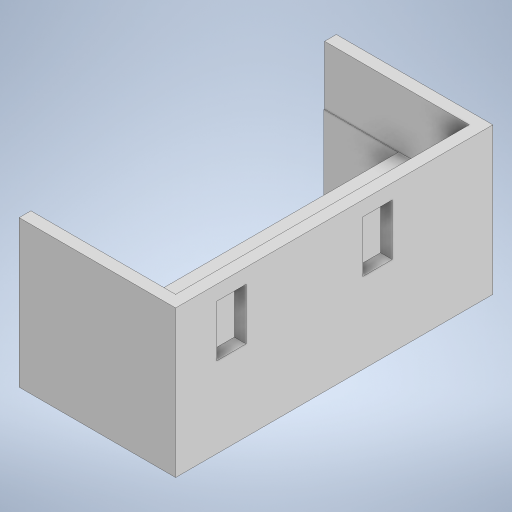
# Autodesk Inventor part: Base1
Saved by Autodesk Inventor 2023 (Build 270158000, 158)
## iProperties
Created: 2022-05-16
Part Number: Base1
Material: Generic
Document SubType Name: Modeling
Designer: WMGWW
Density: 1 g/cm^3
Appearance: Default
Author: WMGWW
Autodesk Inventor part; units mm, degrees
ref_plane "YZ Plane" through (0, 0, 0) normal (1, 0, 0) x (0, 1, 0)
ref_plane "XZ Plane" through (0, 0, 0) normal (0, 1, 0) x (-1, 0, 0)
ref_plane "XY Plane" through (0, 0, 0) normal (0, 0, 1) x (1, 0, 0)
sketch "Sketch1" plane through (0, 0, 0) normal (0, 1, 0) x (-1, 0, 0)
  line L0 (0, 0) -> (25.4, 0)
  line L1 (25.4, 0) -> (25.4, -127)
  line L2 (25.4, -127) -> (0, -127)
  line L3 (0, -127) -> (0, 0)
  line L4 (30.48, 5.08) -> (-5.08, 5.08)
  line L5 (-5.08, 5.08) -> (-5.08, -132.08)
  line L6 (-5.08, -132.08) -> (30.48, -132.08)
  line L7 (30.48, -132.08) -> (30.48, 5.08)
  dimension "d0" = 25.4
  dimension "d1" = 127
  dimension "d2" = 5.08
  dimension "d3" = 5.08
  dimension "d4" = 5.08
  dimension "d5" = 5.08
  constraints: 16 end point, 4 parallel, 2 horizontal, 2 perpendicular
  measures "d0" distance of L0.start L0.end
  measures "d1" distance of L0.end L1.end
  measures "d2" distance between parallel lines of L4 L0
  measures "d3" distance between parallel lines of L6 L2
  measures "d4" distance between parallel lines of L3 L5
  measures "d5" distance between parallel lines of L7 L1
extrude "Extrusion1" add sketch "Sketch1" along normal blind 38.1
sketch "Sketch2" plane through (0, 38.1, 0) normal (0, 1, 0) x (1, 0, 0)
  line L0 (-30.48, -5.08) -> (5.08, -5.08) projected
  line L1 (5.08, -5.08) -> (-62.5812, -5.08)
  line L2 (-62.5812, -5.08) -> (-62.5812, 0)
  line L3 (-62.5812, 0) -> (0, 0)
  line L4 (-25.4, 127) -> (0, 127) projected
  line L5 (0, 127) -> (-62.5812, 127)
  line L6 (5.08, -5.08) -> (5.08, 132.08) projected
  line L7 (5.08, -5.08) -> (-62.5812, -5.08)
  line L8 (-62.5812, 132.08) -> (5.08, 132.08)
  line L9 (5.08, 132.08) -> (5.08, -5.08)
  line L10 (-62.5812, 132.08) -> (-47.0844, 132.08)
  line L11 (-62.5812, 127) -> (-62.5812, 132.08)
  line L12 (0, 127) -> (0, 0) projected
  line L13 (0, 0) -> (0, 127)
  line L14 (0, 127) -> (-62.5812, 127)
  line L15 (-62.5812, 132.08) -> (3.2473, 132.08)
  line L16 (5.08, 132.08) -> (-30.48, 132.08) projected
  constraints: 24 end point, 3 horizontal, 2 perpendicular, 2 point on line, 1 collinear, 1 parallel
extrude "Extrusion2" add sketch "Sketch2" along normal blind 25.4
sketch "Sketch5" plane through (0, 38.1, 0) normal (0, -1, 0) x (1, 0, 0)
  line L0 (-62.5812, -132.08) -> (-62.5812, -127) projected
  line L1 (-30.48, -132.08) -> (-30.48, 5.08) projected
  line L2 (-62.5812, -132.08) -> (-30.48, -132.08)
  line L3 (-30.48, -132.08) -> (-30.48, -126.7104)
  line L4 (-30.48, -126.7104) -> (-62.5812, -126.7104)
  line L5 (-62.5812, -126.7104) -> (-62.5812, -132.08)
  line L6 (-62.5812, 0) -> (-62.5812, 5.08) projected
  line L7 (-30.48, 5.08) -> (5.08, 5.08) projected
  line L8 (-62.5812, 0) -> (-30.48, 0)
  line L9 (-30.48, 0) -> (-30.48, 5.08)
  line L10 (-30.48, 5.08) -> (-62.5812, 5.08)
  line L11 (-62.5812, 5.08) -> (-62.5812, 0)
  point P0 (0, 0)
  constraints: 16 end point, 4 parallel, 2 horizontal, 2 perpendicular, 1 point on line
extrude "Extrusion3" add sketch "Sketch5" along normal blind 38.1
sketch "Sketch6" plane through (-30.48, 0, 0) normal (-1, 0, 0) x (0, 0, 1)
  line L0 (-25.4, 7.62) -> (-38.1, 7.62)
  line L1 (-38.1, 7.62) -> (-38.1, 29.972)
  line L2 (-38.1, 29.972) -> (-25.4, 29.972)
  line L3 (-25.4, 29.972) -> (-25.4, 7.62)
  line L4 (-126.7104, 0) -> (0, 0) projected
  line L5 (0, 63.5) -> (0, 0) projected
  line L6 (-88.6104, 7.62) -> (-101.3104, 7.62)
  line L7 (-101.3104, 7.62) -> (-101.3104, 29.972)
  line L8 (-101.3104, 29.972) -> (-88.6104, 29.972)
  line L9 (-88.6104, 29.972) -> (-88.6104, 7.62)
  line L10 (-126.7104, 38.1) -> (-126.7104, 0) projected
  point P0 (-25.4, 18.796)
  point P1 (-88.6104, 18.796)
  point P2 (-126.7104, 19.05)
  point P3 (-101.3104, 18.796)
  dimension "d12" = 12.7
  dimension "d13" = 22.352
  dimension "d14" = 7.62
  dimension "d15" = 25.4
  dimension "d16" = 12.7
  dimension "d17" = 22.352
  dimension "d18" = 25.4
  dimension "d19" = 7.62
  constraints: 16 end point, 4 midpoint, 4 parallel, 2 horizontal, 2 perpendicular
  measures "d12" distance of L0.start L0.end
  measures "d13" distance of L0.end L1.end
  measures "d14" distance between parallel lines of L4 L0
  measures "d15" distance from line of L5 point (-25.4, 18.796)
  measures "d16" distance of L6.start L6.end
  measures "d17" distance of L6.end L7.end
  measures "d18" horizontal distance of point (-126.71, 19.05) point (-101.31, 18.796)
  measures "d19" distance between parallel lines of L4 L6
extrude "Extrusion4" cut sketch "Sketch6" against normal blind 12.7
sketch "Sketch7" plane through (0, 0, -127) normal (-1, 0, 0) x (0, 0, 1)
  line L0 (51.0896, 34.798) -> (38.3896, 34.798)
  line L1 (38.3896, 34.798) -> (38.3896, 57.15)
  line L2 (38.3896, 57.15) -> (51.0896, 57.15)
  line L3 (51.0896, 57.15) -> (51.0896, 34.798)
  line L4 (38.3896, 29.972) -> (38.3896, 7.62) projected
  line L5 (0, 63.5) -> (127, 63.5) projected
  line L6 (114.3, 34.798) -> (101.6, 34.798)
  line L7 (101.6, 34.798) -> (101.6, 57.15)
  line L8 (101.6, 57.15) -> (114.3, 57.15)
  line L9 (114.3, 57.15) -> (114.3, 34.798)
  line L10 (101.6, 31.5595) -> (101.6, 9.2075)
  line L11 (101.6, 29.972) -> (101.6, 7.62) projected
  point P0 (127, 0)
  point P1 (51.0896, 45.974)
  point P2 (38.3896, 18.796)
  point P3 (44.7396, 57.15)
  point P4 (114.3, 45.974)
  point P5 (101.6, 20.3835)
  point P6 (107.95, 57.15)
  dimension "d22" = 12.7
  dimension "d23" = 22.352
  dimension "d24" = 0
  dimension "d25" = 6.35
  dimension "d26" = 12.7
  dimension "d27" = 22.352
  dimension "d28" = 0
  dimension "d29" = 6.35
  constraints: 18 end point, 6 midpoint, 4 parallel, 2 horizontal, 2 perpendicular, 1 collinear
  measures "d22" distance of L0.start L0.end
  measures "d23" distance of L0.end L1.end
  measures "d24" distance from line of point (38.39, 18.796) L1
  measures "d25" distance from line of L5 point (44.74, 57.15)
  measures "d26" distance of L6.start L6.end
  measures "d27" distance of L6.end L7.end
  measures "d28" distance from line of point (101.6, 20.383) L7
  measures "d29" distance between parallel lines of L5 L8
extrude "Extrusion5" cut sketch "Sketch7" against normal blind 12.7
body "Solid1"
